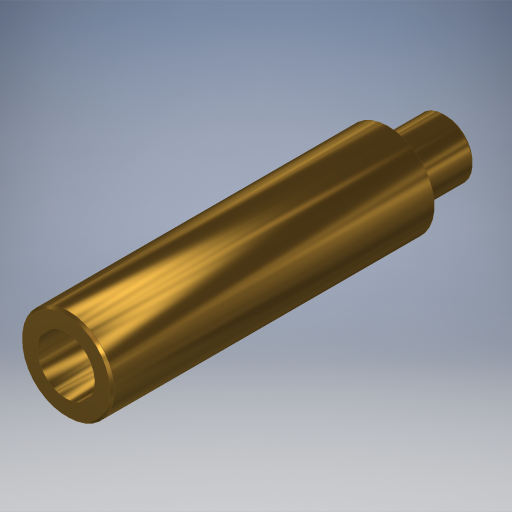
# Autodesk Inventor part: BT805_goteln20_22
Saved by Autodesk Inventor 2023 (Build 270158000, 158)
## iProperties
Company: HTBLA Kaindorf
RuleStatus: InUse
Created: 2023-01-12
Part Number: BT805_goteln20_22
Project: Zeichenmaschine_neu
Material: Messing
Description: getriebe_welle_5zu2
Document SubType Name: Modeling
Designer: goteln20
Density: 8.49 g/cm^3
Appearance: Messing - poliert
Mass: 8.63981 g
Surface Area: 12.9919 cm^2
Volume: 1.01765 cm^3
AfterDocNew0: iProperties-Editor_aufrufen
Author: eligo
Keywords: 22
Autodesk Inventor part; units mm, degrees
ref_plane "YZ Plane" through (0, 0, 0) normal (1, 0, 0) x (0, 1, 0)
ref_plane "XZ Plane" through (0, 0, 0) normal (0, 1, 0) x (-1, 0, 0)
ref_plane "XY Plane" through (0, 0, 0) normal (0, 0, 1) x (1, 0, 0)
sketch "Skizze3" plane through (0, 0, 0) normal (0, 1, 0) x (-1, 0, 0)
  line L0 (-27.6589, 0) -> (27.6589, 0)
  line L1 (-14, 0) -> (-14, 4)
  line L2 (-14, 4) -> (14, 4)
  line L3 (14, 4) -> (14, 2.5)
  line L4 (14, 2.5) -> (19, 2.5)
  line L5 (19, 2.5) -> (19, 0)
  point P0 (0, 0)
  point P1 (0, 0)
  point P2 (14, 3.25)
  point P3 (0, 4)
  dimension "d4" = 8
  dimension "d5" = 5
  dimension "d6" = 5
  dimension "d7" = 28
  constraints: 12 end point, 3 midpoint, 3 perpendicular, 2 horizontal, 2 point on line, 1 coincident, 1 vertical, 1 vertical alignment
  measures "d4" diameter of L2 L0
  measures "d5" diameter of L4 L0
  measures "d6" distance from line of point (14, 3.25) L5
  measures "d7" distance of L1.end L2.end
revolve "Umdrehung1" add sketch "Skizze3" angle 360 about axis through (27.6589, 0, 0) along (-1, 0, 0)
sketch "Skizze4" plane through (14, 0, 0) normal (1, 0, 0) x (0, 0, -1)
  circle A0 centre (0, 0) radius 4 projected
  point P0 (0, 0)
hole "Bohrung1" at (14, 0, 0) direction (-1, 0, 0) diameter 5 depth 22
hole "Bohrung2" at (14, 0, 0) direction (-1, 0, 0) diameter 2 depth 40
sketch "Skizze5" plane through (0, 0, 0) normal (0, 0, 1) x (1, 0, 0)
  line L0 (14, 4) -> (14, -4) projected
  line L1 (-19, 2.5) -> (-19, -2.5) projected
  line L2 (14, 0) -> (-19.3712, 0)
  line L3 (-14, 4) -> (-14, -4) projected
  point P0 (0, 0)
  point P1 (9, 0)
  point P2 (-11, 0)
  dimension "d23" = 3
  dimension "d24" = 5
  constraints: 2 end point, 2 point on line, 1 horizontal, 1 midpoint
  measures "d23" distance from line of L3 point (-11, 0)
  measures "d24" distance from line of L0 point (9, 0)
hole "Bohrung3" at (-11, 0, 0) direction (0, 0, -1) diameter 2 depth 5
hole "Bohrung4" at (9, 0, 0) direction (0, 0, -1) diameter 3 depth 4
thread "Gewinde1" size "M2x0.4" class "6H" standard "ISO Metric profile" length 8
thread "Gewinde2" size "M3x0.5" class "6H" standard "ISO Metric profile" length 8
chamfer "Fase1" distance 0.1 angle 45 4 edges at (9.9974, -1.1203, -3.8399) (9.0005, 1.5, -3.7081) (8.0025, -1.1203, -3.8399) (-11.0007, 1, -3.873)
chamfer "Fase2" distance 0.2 angle 45 2 edges at (14, 0, -4) (-19, 0, -2.5)
